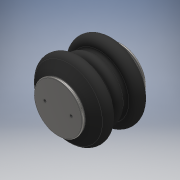
# Autodesk Inventor part: Firestone
Saved by Autodesk Inventor 2018 (Build 220112000, 112)
## iProperties
Created: 2017-11-21
Part Number: Firestone
Material: Rubber
Document SubType Name: Modeling
Designer: P136265
Density: 0.93 g/cm^3
Appearance: Rubber - Black
Author: P136265
Autodesk Inventor part; units mm, degrees
ref_plane "YZ Plane" through (0, 0, 0) normal (1, 0, 0) x (0, 1, 0)
ref_plane "XZ Plane" through (0, 0, 0) normal (0, 1, 0) x (-1, 0, 0)
ref_plane "XY Plane" through (0, 0, 0) normal (0, 0, 1) x (1, 0, 0)
sketch "Sketch1" plane through (0, 0, 0) normal (0, 0, 1) x (1, 0, 0)
  line L0 (0, 0) -> (0, 216)
  line L1 (-126, 0) -> (-126, 216) construction
  line L2 (0, 216) -> (-80, 216)
  line L3 (0, 0) -> (-80, 0)
  line L4 (-80, 216) -> (-80, 0) construction
  line L5 (-126, 108) -> (-80, 108) construction
  line L6 (-126, 216) -> (-80, 216) construction
  line L7 (-103, 216) -> (-103, 108) construction
  line L8 (-126, 0) -> (-80, 0) construction
  line L9 (-103, 0) -> (-103, 108) construction
  arc A0 (-94.4352, 125.906) -> (-94.4352, 90.094) centre (-80, 108) ccw
  arc A1 (-94.4352, 125.906) -> (-100.0909, 139.1847) centre (-99.1423, 131.7449) ccw
  arc A2 (-100.0909, 76.8153) -> (-94.4352, 90.094) centre (-99.1423, 84.2551) ccw
  line L10 (-83, 108) -> (-83, 0) construction
  line L11 (-126, 213) -> (-80, 213) construction
  line L12 (-126, 210) -> (-80, 210) construction
  line L13 (-83, 216) -> (-83, 108) construction
  line L14 (-83, 108) -> (-83, 0) construction
  arc A3 (-80, 216) -> (-80, 210) centre (-80, 213) ccw
  line L15 (-77, 216) -> (-77, 108) construction
  line L16 (-77, 108) -> (-77, 0) construction
  line L17 (-126, 207) -> (-80, 207) construction
  line L18 (-126, 204) -> (-80, 204) construction
  arc A4 (-79.6093, 204.0256) -> (-80, 210) centre (-80, 207) ccw
  line L19 (-80.4259, 203.7277) -> (-115.3877, 181.379)
  arc A5 (-80, 6) -> (-80, 0) centre (-80, 3) ccw
  arc A6 (-80, 6) -> (-79.6093, 11.9744) centre (-80, 9) ccw
  line L20 (-80.4259, 12.2723) -> (-115.3877, 34.621)
  arc A7 (-100.0909, 76.8153) -> (-115.3877, 34.621) centre (-103, 54) ccw
  arc A8 (-115.3877, 181.379) -> (-100.0909, 139.1847) centre (-103, 162) ccw
  arc A9 (-79.6093, 204.0256) -> (-80.4259, 203.7277) centre (-79.3488, 202.0426) ccw
  arc A10 (-80.4259, 12.2723) -> (-79.6093, 11.9744) centre (-79.3488, 13.9574) ccw
  point P0 (-80, 12)
  dimension "d0" = 216
  dimension "d1" = 126
  dimension "d2" = 80
  dimension "d3" = 80
  dimension "d4" = 15
  dimension "d5" = 15
  dimension "d10" = 105
  dimension "d11" = 3
  dimension "d12" = 20
  dimension "d13" = 6
  dimension "d14" = 6
  dimension "d15" = 3
  dimension "d16" = 0
  dimension "d17" = 108
  dimension "d18" = 216
  dimension "d19" = 80
  dimension "d20" = 80
  dimension "d21" = 0
  dimension "d22" = 108
  dimension "d23" = 108
  dimension "d24" = 216
  dimension "d25" = 216
  dimension "d26" = 126
  dimension "d27" = 126
  dimension "d28" = 126
  dimension "d29" = 126
  dimension "d30" = 2
  constraints: 42 end point, 25 point on circle, 16 tangent, 11 centre point, 7 midpoint, 5 parallel, 5 symmetric about line, 3 horizontal, 2 point on line, 1 coincident, 1 equal radius, 1 perpendicular, 1 vertical, 4 other
  measures "d0" distance of L0.start L0.end
  measures "d1" distance between parallel lines of L0 L1
  measures "d2" distance of L0.end L2.end
  measures "d3" distance of L0.start L3.end
  measures "d4" diameter of A1
  measures "d5" diameter of A2
  measures "d10" distance between parallel lines of L5 L11
  measures "d11" distance between parallel lines of L11 L12
  measures "d12" distance between parallel lines of L7 L13
  measures "d13" distance between parallel lines of L13 L15
  measures "d14" distance between parallel lines of L11 L17
  measures "d15" distance between parallel lines of L17 L18
  measures "d16" distance from line of L15.start L2
  measures "d17" distance from line of L15.end L2
  measures "d18" distance from line of L16.end L2
  measures "d19" distance from line of L11.end L0
  measures "d20" distance from line of L17.end L0
  measures "d21" distance from line of L13.start L2
  measures "d22" distance from line of L13.end L2
  measures "d23" distance from line of L10.start L2
  measures "d24" distance from line of L14.end L2
  measures "d25" distance from line of L10.end L2
  measures "d26" distance from line of L11.start L0
  measures "d27" distance from line of L12.start L0
  measures "d28" distance from line of L17.start L0
  measures "d29" distance from line of L18.start L0
  measures "d30" radius of A9
revolve "Revolution1" add sketch "Sketch1" angle 360 about axis through (0, 0, 0) along (0, 1, 0)
sketch "Sketch2" plane through (0, 216, 0) normal (0, 1, 0) x (1, 0, 0)
  circle A0 centre (0, 0) radius 44.5 construction
  circle A1 centre (-44.5, 0) radius 4 construction
  circle A2 centre (44.5, 0) radius 4 construction
  dimension "d32" = 89
  dimension "d33" = 8
  dimension "d34" = 8
  dimension "d35" = 89
  constraints: 3 centre point, 2 point on circle, 1 coincident, 1 horizontal alignment
  measures "d32" diameter of A0
  measures "d33" diameter of A1
  measures "d34" diameter of A2
  measures "d35" distance of A2.centre A1.centre
hole "Hole1" at (-44.5, 216, 0) at (44.5, 216, 0) direction (0, -1, 0) diameter 8 depth 15 tip angle 118
thread "Thread2" size "M8x1.25" class "6H" standard "ANSI Metric M Profile" full length
thread "Thread3" size "M8x1.25" class "6H" standard "ANSI Metric M Profile" full length
sketch "Sketch3" plane through (0, 0, 0) normal (0, -1, 0) x (1, 0, 0)
  circle A0 centre (0, 0) radius 44.5 construction
  circle A1 centre (-44.5, 0) radius 4 construction
  circle A2 centre (-44.5, 0) radius 4 construction
  circle A3 centre (44.5, 0) radius 4 construction
  dimension "d49" = 89
  dimension "d50" = 8
  dimension "d51" = 89
  constraints: 2 centre point, 2 coincident, 1 equal radius, 1 horizontal alignment, 2 other
  measures "d50" diameter of A2
  measures "d51" distance of A1.centre A3.centre
hole "Hole2" at (-44.5, 0, 0) at (44.5, 0, 0) direction (0, 1, 0) diameter 8 depth 15 tip angle 118
thread "Thread4" size "M8x1.25" class "6H" standard "ANSI Metric M Profile" full length
thread "Thread5" size "M8x1.25" class "6H" standard "ANSI Metric M Profile" full length
sketch "Sketch4" plane through (0, 216, 0) normal (0, 1, 0) x (1, 0, 0)
  circle A0 centre (0, -38.1) radius 9.525 construction
  point P0 (0, 0)
  dimension "d63" = 19.05
  dimension "d64" = 38.1
  constraints: 1 centre point, 1 vertical alignment
  measures "d63" diameter of A0
  measures "d64" distance of point (0, 0) A0.centre
hole "Hole3" at (0, 216, 38.1) direction (0, -1, 0) diameter 19.05 depth 15 tip angle 118
thread "Thread6" size "M20x2.5" class "6H" standard "ANSI Metric M Profile" full length
body "Solid1"
